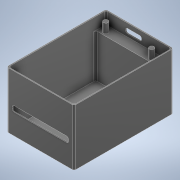
# Autodesk Inventor part: Case - Base
Saved by Autodesk Inventor 2021 (Build 250183000, 183)
## iProperties
Created: 2023-01-24
Part Number: Case - Base
Material: Plástico PC/ABS
Document SubType Name: Modeling
Designer: nicho
Density: 0.357273 g/cm^3
Appearance: Liso - Preto
Author: nicho
Autodesk Inventor part; units mm, degrees
ref_plane "YZ Plane" through (0, 0, 0) normal (1, 0, 0) x (0, 1, 0)
ref_plane "XZ Plane" through (0, 0, 0) normal (0, 1, 0) x (-1, 0, 0)
ref_plane "XY Plane" through (0, 0, 0) normal (0, 0, 1) x (1, 0, 0)
sketch "Esboço1" plane through (0, 0, 0) normal (0, 1, 0) x (-1, 0, 0)
  line L0 (-50, -26.5) -> (50, -26.5)
  line L1 (50, -26.5) -> (50, 26.5)
  line L2 (50, 26.5) -> (-50, 26.5)
  line L3 (-50, 26.5) -> (-50, -26.5)
  line L4 (-50, -26.5) -> (50, 26.5) construction
  line L5 (50, -26.5) -> (-50, 26.5) construction
  point P0 (0, 0)
  dimension "d0" = 100
  dimension "d1" = 53
  constraints: 12 end point, 2 midpoint, 2 parallel, 1 horizontal, 1 perpendicular
  measures "d0" distance of L2.end L1.end
  measures "d1" distance of L1.end L0.end
extrude "Extrusão1" add sketch "Esboço1" along normal blind 30
sketch "Esboço2" plane through (0, 30, 0) normal (0, 1, 0) x (1, 0, 0)
  line L0 (-50, 26.5) -> (-50, -26.5) projected
  line L1 (-50, -26.5) -> (50, -26.5) projected
  line L2 (50, -26.5) -> (50, 26.5) projected
  line L3 (50, 26.5) -> (-50, 26.5) projected
  line L4 (-49.5, -26) -> (-49.5, 26)
  line L5 (-49.5, 26) -> (49.5, 26)
  line L6 (49.5, 26) -> (49.5, -26)
  line L7 (49.5, -26) -> (-49.5, -26)
  point P0 (0, 0)
  dimension "d4" = 0.5
  constraints: 8 end point, 3 other
  measures "d4" distance between parallel lines of L0 L4
extrude "Extrusão2" cut sketch "Esboço2" against normal blind 29.5 contours L4 L5 L6 L7
sketch "Esboço3" plane through (50, 0, -26.5) normal (0, 0, -1) x (-1, 0, 0)
  line L0 (89, 27.5) -> (80.5, 27.5)
  line L1 (80.5, 27.5) -> (80.5, 25)
  line L2 (80.5, 25) -> (89, 25)
  line L3 (89, 25) -> (89, 27.5)
  line L4 (100, 0) -> (100, 30) projected
  line L5 (0, 30) -> (100, 30) projected
  point P0 (50, 0)
  dimension "d7" = 11
  dimension "d8" = 19.5
  dimension "d9" = 2.5
  dimension "d10" = 2.5
  constraints: 8 end point, 2 parallel, 1 horizontal, 1 perpendicular
  measures "d7" distance between parallel lines of L4 L3
  measures "d8" distance between parallel lines of L4 L1
  measures "d9" distance between parallel lines of L0 L2
  measures "d10" distance between parallel lines of L5 L0
extrude "Extrusão3" cut sketch "Esboço3" against normal up to surface (52.5 mm away)
fillet "Arredondamento1" radius 1 4 edges at (-39, 25, -26.25) (-39, 27.5, -26.25) (-30.5, 27.5, -26.25) (-30.5, 25, -26.25)
sketch "Esboço4" plane through (0, 0.5, 0) normal (0, 1, 0) x (1, 0, 0)
  line L0 (-49.5, 26) -> (49.5, 26) projected
  line L1 (-49.5, 26) -> (-18, 26)
  line L2 (-18, 26) -> (-18, 20.5)
  line L3 (-18, 20.5) -> (-49.5, 20.5)
  line L4 (-49.5, 20.5) -> (-49.5, 26)
  point P0 (0, 0)
  dimension "d15" = 5.5
  dimension "d16" = 31.5
  constraints: 8 end point, 2 parallel, 1 horizontal, 1 perpendicular
  measures "d15" distance of L1.end L2.end
  measures "d16" distance of L2.end L3.end
extrude "Extrusão4" add sketch "Esboço4" along normal blind 23
sketch "Esboço5" plane through (0, 23.5, 0) normal (0, 1, 0) x (1, 0, 0)
  circle A0 centre (-46.079, 22.5) radius 1.25
  line L0 (-49.5, -26) -> (-49.5, 26) projected
  line L1 (-49.5, 26) -> (49.5, 26) projected
  circle A1 centre (-21.579, 22.5) radius 1.25
  point P0 (0, 0)
  dimension "d19" = 3.421
  dimension "d20" = 3.5
  dimension "d21" = 2.5
  dimension "d22" = 2.5
  dimension "d23" = 24.5
  constraints: 2 centre point, 1 horizontal alignment
  measures "d19" distance from line of L0 A0.centre
  measures "d20" distance from line of L1 A0.centre
  measures "d21" diameter of A0
  measures "d22" diameter of A1
  measures "d23" distance of A1.centre A0.centre
extrude "Extrusão5" add sketch "Esboço5" along normal blind 5
sketch "Esboço6" plane through (-50, 0, 26.5) normal (0, 0, 1) x (1, 0, 0)
  line L0 (3, 11) -> (33, 11)
  line L1 (33, 11) -> (33, 14)
  line L2 (33, 14) -> (3, 14)
  line L3 (3, 14) -> (3, 11)
  line L4 (0, 0) -> (100, 0) projected
  line L5 (0, 0) -> (0, 30) projected
  point P0 (50, 0)
  dimension "d26" = 11
  dimension "d27" = 14
  dimension "d28" = 30
  dimension "d29" = 3
  constraints: 8 end point, 2 parallel, 1 horizontal, 1 perpendicular
  measures "d26" distance between parallel lines of L0 L4
  measures "d27" distance between parallel lines of L4 L2
  measures "d28" distance of L0.start L0.end
  measures "d29" distance between parallel lines of L5 L3
extrude "Extrusão6" cut sketch "Esboço6" against normal up to surface (47 mm away)
sketch "Esboço7" plane through (-50, 0, 26.5) normal (0, 0, 1) x (1, 0, 0)
  line L0 (0, 30) -> (100, 30) projected
  line L1 (100, 30) -> (36, 30)
  line L2 (36, 30) -> (36, 0)
  line L3 (36, 0) -> (100, 0)
  line L4 (100, 0) -> (100, 30)
  line L5 (33, 14) -> (33, 11) projected
  point P0 (50, 0)
  point P1 (36, 30)
  dimension "d32" = 3
  constraints: 8 end point, 2 parallel, 1 coincident, 1 horizontal, 1 perpendicular
  measures "d32" distance between parallel lines of L5 L2
extrude "Extrusão7" cut sketch "Esboço7" against normal up to surface (53 mm away)
sketch "Esboço8" plane through (0, 0.5, 0) normal (0, 1, 0) x (1, 0, 0)
  line L0 (-14.5, 26) -> (-14.5, -26)
  line L1 (-14, -26) -> (-14, 26) projected
  line L2 (-14, -26) -> (-49.5, -26) projected
  line L3 (-49.5, 26) -> (-14, 26) projected
  point P0 (0, 0)
  dimension "d35" = 0.5
  constraints: 2 end point, 2 point on line, 1 vertical alignment
  measures "d35" distance between parallel lines of L1 L0
extrude "Extrusão8" add sketch "Esboço8" along normal up to surface (29.5 mm away)
fillet "Arredondamento3" radius 1 11 edges at (-14, 15, 26.5) (-14, 15, -26.5) (-49.5, 12, -20.5) (-49.5, 26.75, -26) (-49.5, 15.25, 26) (-50, 15, -26.5) (-14.5, 15.25, 26) (-50, 15, 26.5) (-14.5, 15.25, -26) (-18, 12, -20.5) (-18, 12, -26)
fillet "Arredondamento4" radius 1 4 edges at (-47, 11, 26.25) (-47, 14, 26.25) (-17, 14, 26.25) (-17, 11, 26.25)
